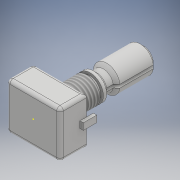
# Autodesk Inventor part: stepped-encoder
Saved by Autodesk Inventor 2018 (Build 220112000, 112)
## iProperties
Created: 2017-11-23
Part Number: stepped-encoder
Material: Generic
Document SubType Name: Modeling
Designer: leo2a
Density: 1 g/cm^3
Appearance: Default
Author: leo2a
Autodesk Inventor part; units mm, degrees
ref_plane "YZ Plane" through (0, 0, 0) normal (1, 0, 0) x (0, 1, 0)
ref_plane "XZ Plane" through (0, 0, 0) normal (0, 1, 0) x (-1, 0, 0)
ref_plane "XY Plane" through (0, 0, 0) normal (0, 0, 1) x (1, 0, 0)
sketch "Sketch1" plane through (0, 0, 0) normal (0, 1, 0) x (-1, 0, 0)
  line L0 (-6.35, 5.5563) -> (-6.35, -5.5563)
  line L1 (-6.35, -5.5563) -> (6.35, -5.5563)
  line L2 (6.35, -5.5563) -> (6.35, 5.5563)
  line L3 (6.35, 5.5563) -> (-6.35, 5.5563)
  line L4 (-6.35, 5.5563) -> (6.35, -5.5563) construction
  line L5 (-6.35, -5.5563) -> (6.35, 5.5563) construction
  point P0 (0, 0)
  dimension "d0" = 11.1125
  dimension "d1" = 12.7
  constraints: 12 end point, 2 midpoint, 2 parallel, 1 perpendicular, 1 vertical
  measures "d0" distance of L0.start L0.end
  measures "d1" distance of L1.end L0.end
extrude "Extrusion1" add sketch "Sketch1" along normal blind 6.35
sketch "Sketch3" plane through (0, 6.35, 0) normal (0, 1, 0) x (1, 0, 0)
  circle A0 centre (0, 0) radius 3.175
  dimension "d8" = 6.35
  constraints: 1 centre point, 1 coincident
  measures "d8" diameter of A0
extrude "Extrusion3" add sketch "Sketch3" along normal blind 6.35
thread "Thread1" size "1/4-32 UNEF" class "2A" standard "ANSI Unified Screw Threads" full length
sketch "Sketch4" plane through (6.35, 0, 5.5563) normal (1, 0, 0) x (0, 0, -1)
  line L0 (4.7625, 4.7625) -> (6.35, 4.7625)
  line L1 (6.35, 4.7625) -> (6.35, 7.9375)
  line L2 (6.35, 7.9375) -> (4.7625, 7.9375)
  line L3 (4.7625, 7.9375) -> (4.7625, 4.7625)
  line L4 (0, 6.35) -> (11.1125, 6.35) projected
  line L5 (4.7625, 4.7625) -> (6.35, 7.9375) construction
  line L6 (6.35, 4.7625) -> (4.7625, 7.9375) construction
  point P0 (5.5563, 0)
  point P1 (5.5563, 6.35)
  dimension "d13" = 1.5875
  dimension "d14" = 3.175
  constraints: 12 end point, 3 midpoint, 2 parallel, 1 perpendicular
  measures "d13" distance of L0.start L0.end
  measures "d14" distance of L1.end L0.end
extrude "Extrusion4" add sketch "Sketch4" along normal blind 0.7937
sketch "Sketch5" plane through (0, 12.7, 0) normal (0, 1, 0) x (1, 0, 0)
  circle A0 centre (0, 0) radius 2.54
  dimension "d17" = 5.08
  constraints: 1 centre point, 1 coincident
  measures "d17" diameter of A0
extrude "Extrusion5" add sketch "Sketch5" along normal blind 0.7937
sketch "Sketch6" plane through (0, 13.4938, 0) normal (0, 1, 0) x (1, 0, 0)
  circle A0 centre (0, 0) radius 3.175
  constraints: 1 centre point, 1 coincident
extrude "Extrusion6" add sketch "Sketch6" along normal blind 12.7
sketch "Sketch7" plane through (0, 26.1938, 0) normal (0, 1, 0) x (1, 0, 0)
  line L0 (-3.175, -0.3969) -> (3.175, -0.3969)
  line L1 (3.175, -0.3969) -> (3.175, 0.3969)
  line L2 (3.175, 0.3969) -> (-3.175, 0.3969)
  line L3 (-3.175, 0.3969) -> (-3.175, -0.3969)
  line L4 (-3.175, -0.3969) -> (3.175, 0.3969) construction
  line L5 (3.175, -0.3969) -> (-3.175, 0.3969) construction
  point P0 (0, 0)
  dimension "d22" = 0.7937
  constraints: 12 end point, 2 midpoint, 2 parallel, 1 horizontal, 1 perpendicular
  measures "d22" distance of L1.end L0.end
extrude "Extrusion7" cut sketch "Sketch7" against normal blind 11.1125
sketch "Sketch8" plane through (3.1501, 26.1938, 0.3969) normal (0, 0, -1) x (-1, 0, 0)
  point P0 (3.1501, -26.1938)
sketch "Sketch9" plane through (0, 15.0813, 0) normal (0, 1, 0) x (1, 0, 0)
  circle A0 centre (0, 0) radius 3.175
  circle A1 centre (0, 0) radius 2.3813
  dimension "d25" = 4.7625
  constraints: 2 centre point, 2 coincident
  measures "d25" diameter of A1
extrude "Extrusion8" cut sketch "Sketch9" along normal blind 1.5875
chamfer "Chamfer1" distance 0.7937 angle 45 3 edges at (0, 16.6687, 3.175) (0, 16.6687, -3.175) (-3.175, 15.0813, 0)
chamfer "Chamfer2" distance 0.7937 angle 45 2 edges at (0, 26.1938, 3.175) (0, 26.1938, -3.175)
fillet "Fillet1" radius 0.7937 11 edges at (0, 6.35, -5.5563) (-6.35, 6.35, 0) (-6.35, 3.175, -5.5563) (0, 0, -5.5563) (6.35, 0, 0) (6.35, 3.175, 5.5563) (0, 6.35, 5.5563) (6.35, 3.175, -5.5563) (0, 0, 5.5563) (-6.35, 3.175, 5.5563) (-6.35, 0, 0)
body "Solid1"
